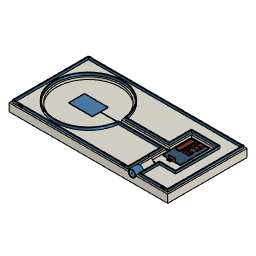
inside (Autodesk Fusion 360 design; units mm, degrees)
Autodesk Fusion 360 part; units mm, degrees
note: some values were not read from the file. Set by a fixed rule: which face or edge a step refers to.
sketch "Sketch1" plane through (0, 0, 0) normal (0, 0, 1) x (1, 0, 0)
  line L0 (-10, 5) -> (10, 5)
  line L1 (10, 5) -> (10, -5)
  line L2 (10, -5) -> (-10, -5)
  line L3 (-10, -5) -> (-10, 5)
  constraint horizontal L0
  constraint vertical L1
  constraint horizontal L2
  constraint vertical L3
extrude "Extrude1" add sketch "Sketch1" along normal blind 1 contours L0 L1 L2 L3 picked at (-3.333333, -1.666667) makes body 1
sketch "Sketch2" plane through (0, 0, 1) normal (0, 0, 1) x (-1, 0, 0)
  line L0 (10, 5) -> (-10, 5)
  line L1 (-10, 5) -> (-10, -5)
  line L2 (-10, -5) -> (10, -5)
  line L3 (10, -5) -> (10, 5)
  circle A0 centre (5, 0) radius 4
  line L4 (-5, -3) -> (-8, -3)
  line L5 (-8, -3) -> (-8, 2)
  line L6 (-8, 2) -> (-5, 2)
  line L7 (-5, 2) -> (-5, -3)
  line L8 (3.5, -0.2) -> (-5, -0.2)
  line L9 (-5, -0.2) -> (-5, 0.2)
  line L10 (-5, 0.2) -> (3.5, 0.2)
  line L11 (3.5, 0.2) -> (3.5, -0.2)
  constraint horizontal L4
  constraint vertical L5
  constraint horizontal L6
  constraint vertical L7
  constraint horizontal L8
  constraint vertical L9
  constraint horizontal L10
  constraint vertical L11
  constraint coincident L7 L9.end
sketch "Sketch3" plane through (0, -5, 0) normal (0, -1, 0) x (1, 0, 0)
  line L0 (-10, 0) -> (10, 0)
  line L1 (10, 0) -> (10, 1)
  line L2 (10, 1) -> (-10, 1)
  line L3 (-10, 1) -> (-10, 0)
  circle A0 centre (5.49068, 1) radius 0.470056
extrude "Extrude2" cut sketch "Sketch2" against normal blind 0.3 contours A0 L8 L10 L11 | A0 L7 L8 L9 L10 | L4 L5 L6 L7 L9 picked at (7.152244, 0.262249) picked at (-2.999815, 0.02223) picked at (-7, -0.4) bodies 1
extrude "Extrude3" cut 1 faces at (-2.666852, 0.02223, 1) along direction (0, 0, -1) blind 0.3 on bodies 1 bodies 1
extrude "Extrude4" cut sketch "Sketch3" against normal blind 3 contours L2 A0 picked at (5.63881, 0.885833) bodies 1
sketch "Sketch4" plane through (0, 0, 0.7) normal (0, 0, 1) x (-1, 0, 0)
  arc A0 (1.005003, -0.2) -> (1.005003, 0.2) centre (5, 0) ccw
  line L0 (1.005003, 0.2) -> (-5, 0.2)
  line L1 (-5, 0.2) -> (-5, 2)
  line L2 (-5, 2) -> (-5.128807, 2)
  line L3 (-5.128807, 2) -> (-5.852553, 2)
  line L4 (-5.852553, 2) -> (-8, 2)
  line L5 (-8, 2) -> (-8, -3)
  line L6 (-8, -3) -> (-5, -3)
  line L7 (-5, -3) -> (-5, -0.2)
  line L8 (-5, -0.2) -> (1.005003, -0.2)
  line L9 (-5.2, -2.8) -> (-7.4, -2.8)
  line L10 (-7.4, -2.8) -> (-7.4, 0.8)
  line L11 (-7.4, 0.8) -> (-5.2, 0.8)
  line L12 (-5.2, 0.8) -> (-5.2, -2.8)
  constraint horizontal L9
  constraint vertical L10
  constraint horizontal L11
  constraint vertical L12
extrude "Extrude5" add sketch "Sketch4" along normal blind 0.1 contours L9 L10 L11 L12 picked at (-5.933333, -1.6) bodies 1
sketch "Sketch5" plane through (0, 0, 0.8) normal (0, 0, 1) x (-1, 0, 0)
  line L0 (-5.2, 0.8) -> (-7.4, 0.8)
  line L1 (-7.4, 0.8) -> (-7.4, -2.8)
  line L2 (-7.4, -2.8) -> (-5.2, -2.8)
  line L3 (-5.2, -2.8) -> (-5.2, 0.8)
  line L4 (-5.9, 0.7) -> (-6.7, 0.7)
  line L5 (-6.7, 0.7) -> (-6.7, 0.8)
  line L6 (-6.7, 0.8) -> (-5.9, 0.8)
  line L7 (-5.9, 0.8) -> (-5.9, 0.7)
  constraint horizontal L4
  constraint vertical L5
  constraint horizontal L6
  constraint vertical L7
  constraint coincident L0 L5.end
extrude "Extrude6" add sketch "Sketch5" along normal blind 0.3 contours L0 L4 L5 L6 L7 picked at (-6.433333, 0.766667) bodies 1
sketch "Sketch6" plane through (0, -0.8, 0) normal (0, -1, 0) x (1, 0, 0)
  line L0 (5.2, 0.7) -> (7.4, 0.7)
  line L1 (7.4, 0.7) -> (7.4, 0.8)
  line L2 (7.4, 0.8) -> (6.7, 0.8)
  line L3 (6.7, 0.8) -> (6.7, 1.1)
  line L4 (6.7, 1.1) -> (5.9, 1.1)
  line L5 (5.9, 1.1) -> (5.9, 0.8)
  line L6 (5.9, 0.8) -> (5.2, 0.8)
  line L7 (5.2, 0.8) -> (5.2, 0.7)
  line L8 (6.04, 0.94) -> (6.12, 0.94)
  line L9 (6.12, 0.94) -> (6.12, 0.86)
  line L10 (6.12, 0.86) -> (6.04, 0.86)
  line L11 (6.04, 0.86) -> (6.04, 0.94)
  line L12 (6.17, 0.94) -> (6.25, 0.94)
  line L13 (6.25, 0.94) -> (6.25, 0.86)
  line L14 (6.25, 0.86) -> (6.17, 0.86)
  line L15 (6.17, 0.86) -> (6.17, 0.94)
  line L16 (6.380562, 0.86011) -> (6.300562, 0.86011)
  line L17 (6.430562, 0.94011) -> (6.510562, 0.94011)
  line L18 (6.300562, 0.94011) -> (6.380562, 0.94011)
  line L19 (6.510562, 0.86011) -> (6.430562, 0.86011)
  line L20 (6.380562, 0.94011) -> (6.380562, 0.86011)
  line L21 (6.300562, 0.86011) -> (6.300562, 0.94011)
  line L22 (6.430562, 0.86011) -> (6.430562, 0.94011)
  line L23 (6.510562, 0.94011) -> (6.510562, 0.86011)
  constraint horizontal L8
  constraint vertical L9
  constraint horizontal L10
  constraint vertical L11
  constraint horizontal L12
  constraint vertical L13
  constraint horizontal L14
  constraint vertical L15
  constraint horizontal L18
  constraint vertical L20
  constraint horizontal L16
  constraint vertical L21
  constraint horizontal L17
  constraint vertical L23
  constraint horizontal L19
  constraint vertical L22
extrude "Extrude7" add sketch "Sketch6" along normal blind 0.4 contours L8 L9 L10 L11 | L12 L13 L14 L15 | L16 L18 L20 L21 | L17 L19 L22 L23 picked at (6.066667, 0.913333) picked at (6.196667, 0.913333) picked at (6.353895, 0.886777) picked at (6.457228, 0.913444) bodies 1
sketch "Sketch7" plane through (0, 0, 0.8) normal (0, 0, 1) x (-1, 0, 0)
  line L0 (-6.7, 0.7) -> (-6.7, 0.8)
  line L1 (-6.7, 0.8) -> (-7.4, 0.8)
  line L2 (-7.4, 0.8) -> (-7.4, -2.8)
  line L3 (-7.4, -2.8) -> (-5.2, -2.8)
  line L4 (-5.2, -2.8) -> (-5.2, 0.8)
  line L5 (-5.2, 0.8) -> (-5.9, 0.8)
  line L6 (-5.9, 0.8) -> (-5.9, 0.7)
  line L7 (-5.9, 0.7) -> (-6.7, 0.7)
  line L8 (-5.4, -2.6) -> (-6, -2.6)
  line L9 (-6, -2.6) -> (-6, -0.5)
  line L10 (-6, -0.5) -> (-5.4, -0.5)
  line L11 (-5.4, -0.5) -> (-5.4, -2.6)
  line L12 (-6.5, -2.6) -> (-7, -2.6)
  line L13 (-7, -2.6) -> (-7, -2.1)
  line L14 (-7, -2.1) -> (-6.5, -2.1)
  line L15 (-6.5, -2.1) -> (-6.5, -2.6)
  line L16 (-6.5, -1.9) -> (-7, -1.9)
  line L17 (-7, -1.9) -> (-7, -1.4)
  line L18 (-7, -1.4) -> (-6.5, -1.4)
  line L19 (-6.5, -1.4) -> (-6.5, -1.9)
  line L20 (-6.1, -2.6) -> (-6.3, -2.6)
  line L21 (-6.3, -2.6) -> (-6.3, -1.5)
  line L22 (-6.3, -1.5) -> (-6.1, -1.5)
  line L23 (-6.1, -1.5) -> (-6.1, -2.6)
  line L24 (-6.1, -1.2) -> (-7, -1.2)
  line L25 (-7, -1.2) -> (-7, -1)
  line L26 (-7, -1) -> (-6.1, -1)
  line L27 (-6.1, -1) -> (-6.1, -1.2)
  line L28 (-6.1, -0.9) -> (-7, -0.9)
  line L29 (-7, -0.9) -> (-7, -0.7)
  line L30 (-7, -0.7) -> (-6.1, -0.7)
  line L31 (-6.1, -0.7) -> (-6.1, -0.9)
  constraint horizontal L8
  constraint vertical L9
  constraint horizontal L10
  constraint vertical L11
  constraint horizontal L12
  constraint vertical L13
  constraint horizontal L14
  constraint vertical L15
  constraint horizontal L16
  constraint vertical L17
  constraint horizontal L18
  constraint vertical L19
  constraint horizontal L20
  constraint vertical L21
  constraint horizontal L22
  constraint vertical L23
  constraint horizontal L24
  constraint vertical L25
  constraint horizontal L26
  constraint vertical L27
  constraint horizontal L28
  constraint vertical L29
  constraint horizontal L30
  constraint vertical L31
extrude "Extrude8" add sketch "Sketch7" along normal blind 0.1 contours L20 L21 L22 L23 picked at (-6.166667, -2.233333) bodies 1
sketch "Sketch8" plane through (0, 0, 0.8) normal (0, 0, 1) x (-1, 0, 0)
  line L0 (-6.1, -1.5) -> (-6.1, -2.6)
  line L1 (-6.1, -2.6) -> (-6.3, -2.6)
  line L2 (-6.3, -2.6) -> (-6.3, -1.5)
  line L3 (-6.3, -1.5) -> (-6.1, -1.5)
  line L4 (-6.7, 0.7) -> (-6.7, 0.8)
  line L5 (-6.7, 0.8) -> (-7.4, 0.8)
  line L6 (-7.4, 0.8) -> (-7.4, -2.8)
  line L7 (-7.4, -2.8) -> (-5.2, -2.8)
  line L8 (-5.2, -2.8) -> (-5.2, 0.8)
  line L9 (-5.2, 0.8) -> (-5.9, 0.8)
  line L10 (-5.9, 0.8) -> (-5.9, 0.7)
  line L11 (-5.9, 0.7) -> (-6.7, 0.7)
  line L12 (-5.4, -2.6) -> (-5.9, -2.6)
  line L13 (-5.9, -2.6) -> (-5.9, -0.6)
  line L14 (-5.9, -0.6) -> (-5.4, -0.6)
  line L15 (-5.4, -0.6) -> (-5.4, -2.6)
  constraint horizontal L12
  constraint vertical L13
  constraint horizontal L14
  constraint vertical L15
extrude "Extrude9" add sketch "Sketch8" along normal blind 0.1 contours L12 L13 L14 L15 picked at (-5.566667, -1.933333) bodies 1
sketch "Sketch9" plane through (0, 0, 0.8) normal (0, 0, 1) x (-1, 0, 0)
  line L0 (-5.4, -0.6) -> (-5.4, -2.6)
  line L1 (-5.4, -2.6) -> (-5.9, -2.6)
  line L2 (-5.9, -2.6) -> (-5.9, -0.6)
  line L3 (-5.9, -0.6) -> (-5.4, -0.6)
  line L4 (-6.1, -1.5) -> (-6.1, -2.6)
  line L5 (-6.1, -2.6) -> (-6.3, -2.6)
  line L6 (-6.3, -2.6) -> (-6.3, -1.5)
  line L7 (-6.3, -1.5) -> (-6.1, -1.5)
  line L8 (-6.7, 0.7) -> (-6.7, 0.8)
  line L9 (-6.7, 0.8) -> (-7.4, 0.8)
  line L10 (-7.4, 0.8) -> (-7.4, -2.8)
  line L11 (-7.4, -2.8) -> (-5.2, -2.8)
  line L12 (-5.2, -2.8) -> (-5.2, 0.8)
  line L13 (-5.2, 0.8) -> (-5.9, 0.8)
  line L14 (-5.9, 0.8) -> (-5.9, 0.7)
  line L15 (-5.9, 0.7) -> (-6.7, 0.7)
  line L16 (-6.5, -2.6) -> (-7, -2.6)
  line L17 (-7, -2.6) -> (-7, -2.2)
  line L18 (-7, -2.2) -> (-6.5, -2.2)
  line L19 (-6.5, -2.2) -> (-6.5, -2.6)
  line L20 (-6.5, -2.1) -> (-7, -2.1)
  line L21 (-7, -2.1) -> (-7, -1.7)
  line L22 (-7, -1.7) -> (-6.5, -1.7)
  line L23 (-6.5, -1.7) -> (-6.5, -2.1)
  line L24 (-6.1, -1.2) -> (-7, -1.2)
  line L25 (-7, -1.2) -> (-7, -1)
  line L26 (-7, -1) -> (-6.1, -1)
  line L27 (-6.1, -1) -> (-6.1, -1.2)
  line L28 (-6.1, -0.9) -> (-7, -0.9)
  line L29 (-7, -0.9) -> (-7, -0.7)
  line L30 (-7, -0.7) -> (-6.1, -0.7)
  line L31 (-6.1, -0.7) -> (-6.1, -0.9)
  constraint horizontal L16
  constraint vertical L17
  constraint horizontal L18
  constraint vertical L19
  constraint horizontal L20
  constraint vertical L21
  constraint horizontal L22
  constraint vertical L23
  constraint horizontal L24
  constraint vertical L25
  constraint horizontal L26
  constraint vertical L27
  constraint horizontal L28
  constraint vertical L29
  constraint horizontal L30
  constraint vertical L31
extrude "Extrude10" add sketch "Sketch9" along normal blind 0.2 contours L16 L17 L18 L19 | L20 L21 L22 L23 | L24 L25 L26 L27 | L28 L29 L30 L31 picked at (-6.666667, -2.466667) picked at (-6.666667, -1.966667) picked at (-6.4, -1.133333) picked at (-6.4, -0.833333) bodies 1
sketch "Sketch10" plane through (0, 0, 0.8) normal (0, 0, 1) x (-1, 0, 0)
  line L0 (-6.1, -0.7) -> (-6.1, -0.9)
  line L1 (-6.1, -0.9) -> (-7, -0.9)
  line L2 (-7, -0.9) -> (-7, -0.7)
  line L3 (-7, -0.7) -> (-6.1, -0.7)
  line L4 (-6.5, -2.2) -> (-6.5, -2.6)
  line L5 (-6.5, -2.6) -> (-7, -2.6)
  line L6 (-7, -2.6) -> (-7, -2.2)
  line L7 (-7, -2.2) -> (-6.5, -2.2)
  line L8 (-6.1, -1) -> (-6.1, -1.2)
  line L9 (-6.1, -1.2) -> (-7, -1.2)
  line L10 (-7, -1.2) -> (-7, -1)
  line L11 (-7, -1) -> (-6.1, -1)
  line L12 (-6.5, -1.7) -> (-6.5, -2.1)
  line L13 (-6.5, -2.1) -> (-7, -2.1)
  line L14 (-7, -2.1) -> (-7, -1.7)
  line L15 (-7, -1.7) -> (-6.5, -1.7)
  line L16 (-5.4, -0.6) -> (-5.4, -2.6)
  line L17 (-5.4, -2.6) -> (-5.9, -2.6)
  line L18 (-5.9, -2.6) -> (-5.9, -0.6)
  line L19 (-5.9, -0.6) -> (-5.4, -0.6)
  line L20 (-6.1, -1.5) -> (-6.1, -2.6)
  line L21 (-6.1, -2.6) -> (-6.3, -2.6)
  line L22 (-6.3, -2.6) -> (-6.3, -1.5)
  line L23 (-6.3, -1.5) -> (-6.1, -1.5)
  line L24 (-6.7, 0.7) -> (-6.7, 0.8)
  line L25 (-6.7, 0.8) -> (-7.4, 0.8)
  line L26 (-7.4, 0.8) -> (-7.4, -2.8)
  line L27 (-7.4, -2.8) -> (-5.2, -2.8)
  line L28 (-5.2, -2.8) -> (-5.2, 0.8)
  line L29 (-5.2, 0.8) -> (-5.9, 0.8)
  line L30 (-5.9, 0.8) -> (-5.9, 0.7)
  line L31 (-5.9, 0.7) -> (-6.7, 0.7)
  circle A0 centre (-6.75, -1.45) radius 0.15
extrude "Extrude11" add sketch "Sketch10" along normal blind 0.4 contours A0 picked at (-6.791312, -1.421834) bodies 1
sketch "Sketch11" plane through (0, -5, 0) normal (0, -1, 0) x (1, 0, 0)
  arc A0 (5.020625, 1) -> (5.960736, 1) centre (5.49068, 1) ccw
  line L0 (5.020625, 1) -> (-10, 1)
  line L1 (-10, 1) -> (-10, 0)
  line L2 (-10, 0) -> (10, 0)
  line L3 (10, 0) -> (10, 1)
  line L4 (10, 1) -> (5.960736, 1)
  circle A1 centre (5.49068, 1) radius 0.450416
  constraint concentric A0 A1
extrude "Extrude12" add sketch "Sketch11" against normal blind 1 separate body contours A1 picked at (5.639142, 0.818137) makes body 2
sketch "Sketch12" plane through (0, -5, 0) normal (0, -1, 0) x (1, 0, 0)
  circle A0 centre (5.49068, 1) radius 0.450416
  circle A1 centre (5.49068, 1) radius 0.363871
  constraint concentric A0 A1
extrude "Extrude13" cut sketch "Sketch12" against normal blind 0.8 contours A1 picked at (5.319479, 1.088377) bodies 2
sketch "Sketch13" plane through (0, -4.2, 0) normal (0, -1, 0) x (1, 0, 0)
  circle A0 centre (5.49068, 1) radius 0.363871
  circle A1 centre (5.49068, 1) radius 0.054978
  constraint concentric A0 A1
extrude "Extrude14" add sketch "Sketch13" along normal blind 0.8 contours A1 picked at (5.505822, 1.010323) bodies 2
sketch "Sketch14" plane through (0, 0, 0.7) normal (0, 0, 1) x (-1, 0, 0)
  line L0 (-5.2, 0.8) -> (-5.2, -2.8)
  line L1 (-5.2, -2.8) -> (-7.4, -2.8)
  line L2 (-7.4, -2.8) -> (-7.4, 0.8)
  line L3 (-7.4, 0.8) -> (-5.2, 0.8)
  arc A0 (1.005003, -0.2) -> (1.005003, 0.2) centre (5, 0) ccw
  line L4 (1.005003, 0.2) -> (-5, 0.2)
  line L5 (-5, 0.2) -> (-5, 2)
  line L6 (-5, 2) -> (-5.128807, 2)
  line L7 (-5.128807, 2) -> (-5.852553, 2)
  line L8 (-5.852553, 2) -> (-8, 2)
  line L9 (-8, 2) -> (-8, -3)
  line L10 (-8, -3) -> (-5, -3)
  line L11 (-5, -3) -> (-5, -0.2)
  line L12 (-5, -0.2) -> (1.005003, -0.2)
  line L13 (6.5, -1) -> (3.5, -1)
  line L14 (3.5, -1) -> (3.5, 1)
  line L15 (3.5, 1) -> (6.5, 1)
  line L16 (6.5, 1) -> (6.5, -1)
  constraint horizontal L13
  constraint vertical L14
  constraint horizontal L15
  constraint vertical L16
extrude "Extrude15" add sketch "Sketch14" along normal blind 0.05 contours L13 L14 L15 L16 picked at (5.5, -0.333333) bodies 1
sketch "Sketch15" plane through (0, 0, 0.7) normal (0, 0, 1) x (-1, 0, 0)
  line L0 (6.5, 1) -> (6.5, -1)
  line L1 (6.5, -1) -> (3.5, -1)
  line L2 (3.5, -1) -> (3.5, 1)
  line L3 (3.5, 1) -> (6.5, 1)
  line L4 (-5.2, 0.8) -> (-5.2, -2.8)
  line L5 (-5.2, -2.8) -> (-7.4, -2.8)
  line L6 (-7.4, -2.8) -> (-7.4, 0.8)
  line L7 (-7.4, 0.8) -> (-5.2, 0.8)
  arc A0 (1.005003, -0.2) -> (1.005003, 0.2) centre (5, 0) ccw
  line L8 (1.005003, 0.2) -> (-5, 0.2)
  line L9 (-5, 0.2) -> (-5, 2)
  line L10 (-5, 2) -> (-5.128807, 2)
  line L11 (-5.128807, 2) -> (-5.852553, 2)
  line L12 (-5.852553, 2) -> (-8, 2)
  line L13 (-8, 2) -> (-8, -3)
  line L14 (-8, -3) -> (-5, -3)
  line L15 (-5, -3) -> (-5, -0.2)
  line L16 (-5, -0.2) -> (1.005003, -0.2)
  line L17 (3.5, 0) -> (-5.2, 0)
  line L18 (-5.2, 0) -> (-5.2, -0.020037)
  line L19 (-5.2, -0.020037) -> (3.5, -0.020037)
  line L20 (3.5, -0.020037) -> (3.5, 0)
  constraint horizontal L17
  constraint vertical L18
  constraint horizontal L19
  constraint vertical L20
  constraint midpoint L2 L17.start
extrude "Extrude16" add sketch "Sketch15" along normal blind 0.05 separate body contours L2 L4 L17 L18 L19 L20 picked at (-2.3, -0.006679) makes body 3
sketch "Sketch16" plane through (0, 0, 1) normal (0, 0, 1) x (-1, 0, 0)
  line L0 (-5.020625, 5) -> (-5.020625, 2)
  line L1 (-5.020625, 2) -> (-5, 2)
  line L2 (-5, 2) -> (-5, 0.2)
  line L3 (-5, 0.2) -> (1.005003, 0.2)
  arc A0 (1.005003, -0.2) -> (1.005003, 0.2) centre (5, 0) ccw
  line L4 (1.005003, -0.2) -> (-5, -0.2)
  line L5 (-5, -0.2) -> (-5, -3)
  line L6 (-5, -3) -> (-8, -3)
  line L7 (-8, -3) -> (-8, 2)
  line L8 (-8, 2) -> (-5.960736, 2)
  line L9 (-5.960736, 2) -> (-5.960736, 5)
  line L10 (-5.960736, 5) -> (-10, 5)
  line L11 (-10, 5) -> (-10, -5)
  line L12 (-10, -5) -> (10, -5)
  line L13 (10, -5) -> (10, 5)
  line L14 (10, 5) -> (-5.020625, 5)
  line L15 (9.8, 4.8) -> (-4.820625, 4.8)
  line L16 (-4.820625, 4.8) -> (-4.820625, 2.2)
  line L17 (-4.820625, 2.2) -> (-4.8, 2.2)
  line L18 (-4.8, 2.2) -> (-4.8, 0.4)
  line L19 (-4.8, 0.4) -> (0.819091, 0.4)
  arc A1 (0.819091, -0.4) -> (0.819091, 0.4) centre (5, 0) ccw
  line L20 (0.819091, -0.4) -> (-4.8, -0.4)
  line L21 (-4.8, -0.4) -> (-4.8, -3.2)
  line L22 (-4.8, -3.2) -> (-8.2, -3.2)
  line L23 (-8.2, -3.2) -> (-8.2, 2.2)
  line L24 (-8.2, 2.2) -> (-6.160736, 2.2)
  line L25 (-6.160736, 2.2) -> (-6.160736, 4.8)
  line L26 (-6.160736, 4.8) -> (-9.8, 4.8)
  line L27 (-9.8, 4.8) -> (-9.8, -4.8)
  line L28 (-9.8, -4.8) -> (9.8, -4.8)
  line L29 (9.8, -4.8) -> (9.8, 4.8)
  line L30 (9.7, 4.7) -> (-4.720625, 4.7)
  line L31 (-4.720625, 4.7) -> (-4.720625, 2.299999)
  line L32 (-4.720625, 2.299999) -> (-4.7, 2.299999)
  line L33 (-4.7, 2.299999) -> (-4.7, 0.5)
  line L34 (-4.7, 0.5) -> (0.729169, 0.5)
  arc A2 (0.729169, -0.5) -> (0.729169, 0.5) centre (5, 0) ccw
  line L35 (0.729169, -0.5) -> (-4.7, -0.5)
  line L36 (-4.7, -0.5) -> (-4.7, -3.3)
  line L37 (-4.7, -3.3) -> (-8.3, -3.3)
  line L38 (-8.3, -3.3) -> (-8.3, 2.3)
  line L39 (-8.3, 2.3) -> (-6.260736, 2.3)
  line L40 (-6.260736, 2.3) -> (-6.260736, 4.7)
  line L41 (-6.260736, 4.7) -> (-9.7, 4.7)
  line L42 (-9.7, 4.7) -> (-9.7, -4.7)
  line L43 (-9.7, -4.7) -> (9.7, -4.7)
  line L44 (9.7, -4.7) -> (9.7, 4.7)
  dimension "d33" = -0.2
  dimension "d34" = -0.3
extrude "Extrude17" add sketch "Sketch16" along normal blind 0.3 separate body contours L15 L16 L17 L18 L19 A1 L20 L21 L22 L23 L24 L25 L26 L27 L28 L29 picked at (0.824215, 0.638191) makes body 4
sketch "Sketch17" plane through (0, -4.8, 0) normal (0, -1, 0) x (1, 0, 0)
  line L0 (-9.8, 1) -> (4.820625, 1)
  line L1 (4.820625, 1) -> (4.820625, 1.3)
  line L2 (4.820625, 1.3) -> (-9.8, 1.3)
  line L3 (-9.8, 1.3) -> (-9.8, 1)
  line L4 (-8.991827, 1.213831) -> (-8.499071, 1.213831)
  line L5 (-8.499071, 1.213831) -> (-8.499071, 1.153398)
  line L6 (-8.499071, 1.153398) -> (-8.991827, 1.153398)
  line L7 (-8.991827, 1.153398) -> (-8.991827, 1.213831)
  line L8 (3.991804, 1.195236) -> (4.489208, 1.195236)
  line L9 (4.489208, 1.195236) -> (4.489208, 1.120858)
  line L10 (4.489208, 1.120858) -> (3.991804, 1.120858)
  line L11 (3.991804, 1.120858) -> (3.991804, 1.195236)
  constraint horizontal L4
  constraint vertical L5
  constraint horizontal L6
  constraint vertical L7
  constraint horizontal L8
  constraint vertical L9
  constraint horizontal L10
  constraint vertical L11
extrude "Extrude18" add sketch "Sketch17" along normal blind 0.1 contours L4 L5 L6 L7 picked at (-8.663323, 1.173542) bodies 4
extrude "Extrude19" add sketch "Sketch17" along normal blind 0.1 contours L8 L9 L10 L11 picked at (4.157606, 1.170443) bodies 4
sketch "Sketch18" plane through (0, -4.8, 0) normal (0, -1, 0) x (1, 0, 0)
  line L0 (6.160736, 1) -> (9.8, 1)
  line L1 (9.8, 1) -> (9.8, 1.3)
  line L2 (9.8, 1.3) -> (6.160736, 1.3)
  line L3 (6.160736, 1.3) -> (6.160736, 1)
  line L4 (8.997964, 1.246412) -> (9.497603, 1.246412)
  line L5 (9.497603, 1.246412) -> (9.497603, 1.180367)
  line L6 (9.497603, 1.180367) -> (8.997964, 1.180367)
  line L7 (8.997964, 1.180367) -> (8.997964, 1.246412)
  constraint horizontal L4
  constraint vertical L5
  constraint horizontal L6
  constraint vertical L7
extrude "Extrude20" add sketch "Sketch18" along normal blind 0.1 contours L4 L5 L6 L7 picked at (9.164511, 1.224397) bodies 4
sketch "Sketch19" plane through (0, 4.8, 0) normal (0, 1, 0) x (-1, 0, 0)
  line L0 (-9.8, 1) -> (9.8, 1)
  line L1 (9.8, 1) -> (9.8, 1.3)
  line L2 (9.8, 1.3) -> (-9.8, 1.3)
  line L3 (-9.8, 1.3) -> (-9.8, 1)
  line L4 (-9.755068, 1.245571) -> (-9.499506, 1.245571)
  line L5 (-9.499506, 1.245571) -> (-9.499506, 1.20537)
  line L6 (-9.499506, 1.20537) -> (-9.755068, 1.20537)
  line L7 (-9.755068, 1.20537) -> (-9.755068, 1.245571)
  line L8 (9.503976, 1.242699) -> (9.750924, 1.242699)
  line L9 (9.750924, 1.242699) -> (9.750924, 1.208241)
  line L10 (9.750924, 1.208241) -> (9.503976, 1.208241)
  line L11 (9.503976, 1.208241) -> (9.503976, 1.242699)
  constraint horizontal L4
  constraint vertical L5
  constraint horizontal L6
  constraint vertical L7
  constraint horizontal L8
  constraint vertical L9
  constraint horizontal L10
  constraint vertical L11
extrude "Extrude21" add sketch "Sketch19" along normal blind 0.1 contours L4 L5 L6 L7 picked at (-9.669881, 1.23217) bodies 4
extrude "Extrude22" add sketch "Sketch19" along normal blind 0.1 contours L8 L9 L10 L11 picked at (9.586292, 1.231213) bodies 4
